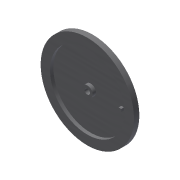
# Autodesk Inventor part: base
Saved by Autodesk Inventor 2022 Beta2 (Build 260130000, 130) ContinuousBuild 0
## iProperties
Shininess: 64.0
Length Units: 11272
Angle Units: 11279
Time Units: 11290
Mass Units: 11286
Length Display Precision: 3
Angle Display Precision: 2
Created: 2002-02-11
Part Number: base
Document SubType Name: Modeling
Designer: Administrator
Density: 1 g/cm^3
Material: Generic
Appearance: Light Gray
Density: 0.0
Volumn: 0.0
Area: 0.0
PropertySet Name: Model Information
Control State: 0
Master: False
Checked Out: False
Author: Administrator
Autodesk Inventor part; units mm, degrees
ref_plane "YZ Plane" through (0, 0, 0) normal (1, 0, 0) x (0, 1, 0)
ref_plane "XZ Plane" through (0, 0, 0) normal (0, 1, 0) x (-1, 0, 0)
ref_plane "XY Plane" through (0, 0, 0) normal (0, 0, 1) x (1, 0, 0)
sketch "Sketch1" plane through (0, 0, 0) normal (0, 0, 1) x (1, 0, 0)
  circle A0 centre (0, 0) radius 111.125
  dimension "d0" = 222.25
  constraints: 1 centre point
  measures "d0" diameter of A0
extrude "Extrusion1" add sketch "Sketch1" along normal blind 12.7
sketch "Sketch2" plane through (0, 0, 12.7) normal (0, 0, 1) x (1, 0, 0)
  circle A0 centre (0, 0) radius 111.125 projected
  circle A1 centre (0, 0) radius 88.9
  circle A2 centre (0, 0) radius 12.7
  dimension "d3" = 177.8
  dimension "d4" = 25.4
  constraints: 2 centre point, 2 coincident
  measures "d3" diameter of A1
  measures "d4" diameter of A2
extrude "Extrusion2" cut sketch "Sketch2" against normal blind 7.9375 contours A1
sketch "Sketch3" plane through (0, 0, 12.7) normal (0, 0, 1) x (1, 0, 0)
  circle A0 centre (0, 0) radius 12.7 projected
hole "Hole1" at (0, 0, 12.7) direction (0, 0, -1) diameter 12.7 end through all
sketch "Sketch4" plane through (0, 0, 4.7625) normal (0, 0, 1) x (1, 0, 0)
  circle A0 centre (0, 0) radius 12.7 projected
  line L0 (73.025, 3.175) -> (79.375, 3.175)
  line L1 (79.375, 3.175) -> (79.375, -3.175)
  line L2 (79.375, -3.175) -> (73.025, -3.175)
  line L3 (73.025, -3.175) -> (73.025, 3.175)
  circle A1 centre (76.2, 0) radius 3.175 construction
  circle A2 centre (0, 0) radius 6.35 projected
  dimension "d14" = 76.2
  dimension "d15" = 6.35
  constraints: 8 end point, 4 tangent, 2 parallel, 1 centre point, 1 horizontal, 1 horizontal alignment, 1 perpendicular
  measures "d14" distance of A1.centre A2.centre
  measures "d15" diameter of A1
extrude "Extrusion3" add sketch "Sketch4" along normal blind 6.6675 contours L0 L1 L2 L3
sketch "Sketch5" plane through (0, 0, 0) normal (0, 0, -1) x (-1, 0, 0)
  circle A0 centre (0, 0) radius 6.35 projected
  circle A1 centre (0, 0) radius 111.125 projected
  circle A2 centre (0, 0) radius 9.525
  dimension "d18" = 19.05
  constraints: 1 centre point, 1 coincident
  measures "d18" diameter of A2
extrude "Extrusion4" cut sketch "Sketch5" against normal blind 3.81 contours A2
body "Solid1"
